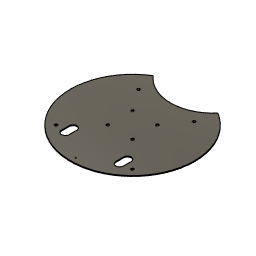
BaseChapaCima (Autodesk Fusion 360 archive; units mm, degrees)
design "Plate_Top"
Autodesk Fusion 360 part; units mm, degrees
sketch "Esboço1" plane through (0, 0, 0) normal (0, 0, 1) x (1, 0, 0)
  circle A0 centre (0, 0) radius 240
  line L0 (48, -48) -> (-48, -48)
  line L1 (-48, -48) -> (-48, 48)
  line L2 (-48, 48) -> (48, 48)
  line L3 (48, 48) -> (48, -48)
  line L4 (48, -48) -> (-48, 48) construction
  line L5 (-48, -48) -> (48, 48) construction
  circle A1 centre (-48, 48) radius 5
  circle A2 centre (-48, -48) radius 5
  circle A3 centre (48, 48) radius 5
  circle A4 centre (48, -48) radius 5
  line L6 (105, -110) -> (105, -170)
  line L7 (90, -125) -> (90, -155)
  line L8 (120, -125) -> (120, -155)
  arc A5 (120, -125) -> (90, -125) centre (105, -125) ccw
  arc A6 (90, -155) -> (120, -155) centre (105, -155) ccw
  circle A7 centre (148, -148) radius 5
  line L9 (-125, 204.878) -> (125, 204.878)
  circle A8 centre (0, 311.043) radius 164
  circle A9 centre (107.5, 130.5) radius 5
  line L10 (-40, 115) -> (40, 115)
  line L11 (-40, 115) -> (-40, 151.9958)
  line L12 (40, 115) -> (40, 151.9958)
  line L13 (0, 1.75) -> (0, 22.5)
  line L14 (-120, -125) -> (-120, -155)
  arc A10 (-90, -125) -> (-120, -125) centre (-105, -125) ccw
  line L15 (-90, -125) -> (-90, -155)
  arc A11 (-120, -155) -> (-90, -155) centre (-105, -155) ccw
  circle A12 centre (-148, -148) radius 5
  circle A13 centre (-107.5, 130.5) radius 5
  circle A14 centre (0, -220) radius 2
  point P0 (105, -110)
  point P1 (0, 115)
  dimension "d1" = 480
  dimension "d2" = 96
  dimension "d3" = 96
  dimension "d4" = 10
  dimension "d5" = 10
  dimension "d6" = 10
  dimension "d7" = 10
  dimension "d8" = 110
  dimension "d9" = 105
  dimension "d10" = 30
  dimension "d11" = 60
  dimension "d12" = 30
  dimension "d13" = 10
  dimension "d14" = 148
  dimension "d15" = 148
  dimension "d16" = 250
  dimension "d17" = 328
  dimension "d18" = 10
  dimension "d19" = 130.5
  dimension "d20" = 107.5
  dimension "d21" = 115
  dimension "d22" = 80
  dimension "d23" = 4
  dimension "d24" = 220
  constraint coincident A0.centre origin
  constraint horizontal L0
  constraint perpendicular L0 L1
  constraint parallel L0 L2
  constraint parallel L1 L3
  constraint coincident L4 A0.centre
  constraint coincident L5 A0.centre
  constraint coincident L1.end L2.start
  constraint coincident L0.end L1.start
  constraint coincident L2.end L3.start
  constraint coincident L0.start L3.end
  constraint coincident P0 A5
  constraint coincident P0 L6.start
  constraint vertical L6
  constraint coincident A5.centre L6
  constraint coincident L6.end A6
  constraint tangent L7 A6
  constraint parallel L6 L7
  constraint tangent L8 A6
  constraint parallel L6 L8
  constraint horizontal L9
  constraint coincident A0 L9.start
  constraint coincident A0 L9.end
  constraint coincident L9.start A8
  constraint coincident L9.end A8
  constraint horizontal L10
  constraint midpoint P1 L10
  constraint coincident A8 L11.end
  constraint perpendicular L10 L11
  constraint coincident A8 L12.end
  constraint perpendicular L10 L12
  constraint symmetric L7.start L13 A10.start
  constraint symmetric L7.end L13 L15.end
  constraint symmetric L8.start L13 L14.start
  constraint symmetric L8.end L13 L14.end
  constraint symmetric A5 L13 A10
  constraint symmetric A6 L13 A11
  constraint symmetric A7 L13 A12
  constraint symmetric A9 L13 A13
  measures "d1" diameter of A0
  measures "d2" distance of L1.end L2.end
  measures "d3" distance of L0.end L1.end
  measures "d4" diameter of A1
  measures "d5" diameter of A2
  measures "d6" diameter of A3
  measures "d7" diameter of A4
  measures "d8" vertical distance of A0.centre P0
  measures "d9" horizontal distance of A0.centre P0
  measures "d10" diameter of A5
  measures "d11" distance of P0 L6.end
  measures "d12" diameter of A6
  measures "d13" diameter of A7
  measures "d14" vertical distance of A0.centre A7.centre
  measures "d15" horizontal distance of A0.centre A7.centre
  measures "d16" distance of L9.start L9.end
  measures "d17" diameter of A8
  measures "d18" diameter of A9
  measures "d19" vertical distance of A0.centre A9.centre
  measures "d20" horizontal distance of A0.centre A9.centre
  measures "d21" distance of A0.centre P1
  measures "d22" distance of L10.start L10.end
  measures "d23" diameter of A14
  measures "d24" distance of A0.centre A14.centre
extrude "Extrusão1" add sketch "Esboço1" along normal blind 3 contours A0 A8 L10 L11 L12 | A8 L10 L11 L12 | L0 L1 L2 L3 A1 A2 A3 A4
equation "d12 = d10"
equation "d17 = ( 164 * 2 ) * 1 mm"
equation "d24 = d1 / 2 - 20 mm"
